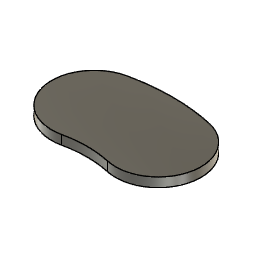
os3m_custom_target_v0 (Autodesk Fusion 360 design; units mm, degrees)
Autodesk Fusion 360 part; units mm, degrees
sketch "Sketch1" plane through (0, 0, 0) normal (0, 0, 1) x (1, 0, 0)
  line L0 (-18.15, -10.4789) -> (0, 20.9578) construction
  line L1 (0, 20.9578) -> (18.15, -10.4789) construction
  line L2 (18.15, -10.4789) -> (-18.15, -10.4789) construction
  circle A0 centre (0, 0) radius 20.9578 construction
  line L3 (4.5, 20.469) -> (-4.5, 20.469) construction
  line L4 (0, 20.469) -> (0, 20.9578) construction
  arc A1 (5.7883, 26.3291) -> (-5.7883, 26.3291) centre (0, 0) ccw
  arc A2 (3.2117, 14.6089) -> (-3.2117, 14.6089) centre (0, 0) ccw
  arc A3 (-5.9382, 20.0989) -> (-2.8501, 26.2377) centre (0, 20.9578) ccw construction
  arc A4 (2.8501, 26.2377) -> (-1.0433, 22.7649) centre (4.5, 20.469) ccw construction
  arc A5 (1.4841, 20.9052) -> (-2.8501, 26.2377) centre (-4.5, 20.469) ccw construction
  arc A6 (-2.8501, 26.2377) -> (-1.6499, 15.1891) centre (-4.5, 20.469) ccw
  arc A7 (0, 16.5004) -> (1.4841, 20.9052) centre (-4.5, 20.469) ccw
  arc A8 (-1.6499, 15.1891) -> (0, 16.5004) centre (-4.5, 20.469) ccw construction
  arc A9 (-1.4841, 20.9052) -> (0, 16.5004) centre (4.5, 20.469) ccw
  arc A10 (1.6499, 15.1891) -> (2.8501, 26.2377) centre (4.5, 20.469) ccw
  arc A11 (0, 16.5004) -> (1.6499, 15.1891) centre (4.5, 20.469) ccw construction
  dimension "d1" = 60
  dimension "d2" = 60
  dimension "d3" = 60
  dimension "d4" = 36.3
  dimension "d5" = 12
  dimension "d7" = 12
  dimension "d8" = 12
  dimension "d9" = 9
  constraint horizontal L2
  constraint coincident L1.end A0
  constraint coincident L0.end A0
  constraint coincident L0.start A0
  constraint coincident A0.centre A1.centre
  constraint coincident L0.end L1.start
  constraint coincident A0 L3.start
  constraint coincident A0 L3.end
  constraint coincident L3.start A4.centre
  constraint coincident L3.end A5.centre
  constraint midpoint L3 L4.start
  constraint vertical L4
  constraint tangent A1 A3
  constraint coincident A1.start A9
  constraint coincident A1.end A6
  constraint tangent A2 A3
  constraint coincident A2.start A9
  constraint coincident A2.end A6
  constraint tangent A2 A9
  constraint tangent A2 A6
  constraint tangent A1 A9
  constraint tangent A1 A6
  constraint coincident A0 A3.start
  constraint coincident A3 A4.start
  constraint coincident A0 A9.start
  constraint concentric A4 A9
  constraint coincident L1 A4.end
  constraint coincident A9.start A4
  constraint coincident A0 A5.start
  constraint concentric A5 A6
  constraint coincident A3 A6.end
  constraint concentric A6 A7
  constraint concentric A6 A8
  constraint coincident A3 A10.start
  constraint concentric A9 A10
  constraint concentric A9 A11
  measures "d1" angle of L1 L2
  measures "d2" angle of L0 L1
  measures "d3" angle of L0 L2
  measures "d4" distance of L0.start L1.end
  measures "d5" diameter of A3
  measures "d7" diameter of A9
  measures "d8" diameter of A6
  measures "d9" horizontal distance of L3.start L3.end
extrude "Extrude1" add sketch "Sketch1" along normal blind 1.3
equation "d5 = coil_dia"
equation "coil_dia = 12 mm"
equation "d7 = coil_dia"
equation "d8 = coil_dia"
equation "d9 = coil_dia * 0.75"
named bodies: "os3m_hypothesis_target"
